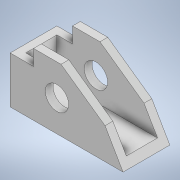
# Autodesk Inventor part: Assignment 1.4 - Guide Block
Saved by Autodesk Inventor 2021.1 (Build 251245000, 245)
## iProperties
Created: 2021-05-13
Part Number: Assignment 1.4 - Guide Block
Material: Generic
Document SubType Name: Modeling
Designer: as000166
Density: 1 g/cm^3
Appearance: Default
Author: as000166
Autodesk Inventor part; units mm, degrees
ref_plane "YZ Plane" through (0, 0, 0) normal (1, 0, 0) x (0, 1, 0)
ref_plane "XZ Plane" through (0, 0, 0) normal (0, 1, 0) x (-1, 0, 0)
ref_plane "XY Plane" through (0, 0, 0) normal (0, 0, 1) x (1, 0, 0)
sketch "Sketch1" plane through (0, 0, 0) normal (0, 0, 1) x (1, 0, 0)
  line L0 (0, 0) -> (91.948, 0)
  line L1 (0, 0) -> (0, 38.1)
  line L2 (0, 38.1) -> (19.05, 38.1)
  line L3 (19.05, 38.1) -> (19.05, 50.8)
  line L4 (19.05, 50.8) -> (41.402, 50.8)
  line L5 (91.948, 0) -> (77.2833, 25.4)
  line L6 (41.402, 50.8) -> (77.2833, 25.4)
  circle A0 centre (38.1, 25.4) radius 9.525
  dimension "d0" = 91.948
  dimension "d1" = 38.1
  dimension "d2" = 19.05
  dimension "d3" = 12.7
  dimension "d4" = 22.352
  dimension "d6" = 60
  dimension "d9" = 19.05
  constraints: 14 end point, 2 perpendicular, 2 vertical, 1 centre point, 1 horizontal
  measures "d0" distance of L0.start L0.end
  measures "d1" distance of L0.start L1.end
  measures "d2" distance of L1.end L2.end
  measures "d3" distance of L2.end L3.end
  measures "d4" distance of L3.end L4.end
  measures "d6" angle of L0 L5
  measures "d9" diameter of A0
extrude "Extrusion5" add sketch "Sketch1" against normal blind 38.1
sketch "Sketch10" plane through (19.05, 50.8, 0) normal (0, 1, 0) x (1, 0, 0)
  line L0 (69.723, 6.3497) -> (69.723, 31.75)
  line L1 (69.723, 31.75) -> (-12.7, 31.75)
  line L2 (-12.7, 31.75) -> (-12.7, 6.3497)
  line L3 (-12.7, 6.3497) -> (69.723, 6.3497)
  point P0 (-19.05, 0)
  constraints: 8 end point, 2 vertical, 1 perpendicular
extrude "Extrusion7" cut sketch "Sketch10" against normal blind 44.45
body "Solid3"
